Autodesk Inventor part; units mm, degrees
(part 2 of 2)
  circle A233 centre (35.381, -14.7938) radius 0.4555 projected
  circle A234 centre (37.921, -17.3338) radius 0.4555 projected
  circle A235 centre (35.381, -17.3338) radius 0.4555 projected
  circle A236 centre (35.381, -19.8738) radius 0.4555 projected
  circle A237 centre (35.381, -22.4138) radius 0.4555 projected
  circle A238 centre (37.921, -19.8738) radius 0.4555 projected
  circle A239 centre (37.921, -24.9538) radius 0.4555 projected
  circle A240 centre (37.921, -22.4138) radius 0.4555 projected
  circle A241 centre (35.381, -24.9538) radius 0.4555 projected
  circle A242 centre (37.921, -27.4938) radius 0.4555 projected
  circle A243 centre (35.381, -27.4938) radius 0.4555 projected
  circle A244 centre (37.921, -30.0338) radius 0.4555 projected
  circle A245 centre (35.381, -30.0338) radius 0.4555 projected
  circle A246 centre (37.921, -32.5738) radius 0.4555 projected
  circle A247 centre (35.381, -32.5738) radius 0.4555 projected
  circle A248 centre (37.921, -35.1138) radius 0.4555 projected
  circle A249 centre (35.381, -35.1138) radius 0.4555 projected
  circle A250 centre (35.381, -37.6538) radius 0.4555 projected
  circle A251 centre (81.101, -12.2538) radius 0.4555 projected
  circle A252 centre (78.561, -32.5738) radius 0.4555 projected
  circle A253 centre (81.101, -32.5738) radius 0.4555 projected
  circle A254 centre (78.561, -30.0338) radius 0.4555 projected
  circle A255 centre (81.101, -30.0338) radius 0.4555 projected
  circle A256 centre (78.561, -27.4938) radius 0.4555 projected
  circle A257 centre (81.101, -27.4938) radius 0.4555 projected
  circle A258 centre (78.561, -24.9538) radius 0.4555 projected
  circle A259 centre (81.101, -24.9538) radius 0.4555 projected
  circle A260 centre (78.561, -22.4138) radius 0.4555 projected
  circle A261 centre (81.101, -22.4138) radius 0.4555 projected
  circle A262 centre (78.561, -19.8738) radius 0.4555 projected
  circle A263 centre (81.101, -19.8738) radius 0.4555 projected
  circle A264 centre (78.561, -17.3338) radius 0.4555 projected
  circle A265 centre (81.101, -17.3338) radius 0.4555 projected
  circle A266 centre (78.561, -14.7938) radius 0.4555 projected
  circle A267 centre (81.101, -14.7938) radius 0.4555 projected
  circle A268 centre (78.561, -12.2538) radius 0.4555 projected
  circle A269 centre (78.561, -9.7138) radius 0.4555 projected
  circle A270 centre (81.101, -9.7138) radius 0.4555 projected
  circle A271 centre (78.561, -7.1738) radius 0.4555 projected
  circle A272 centre (81.101, -7.1738) radius 0.4555 projected
  circle A273 centre (78.561, -4.6338) radius 0.4555 projected
  circle A274 centre (81.101, -4.6338) radius 0.4555 projected
  circle A275 centre (78.561, -2.0938) radius 0.4555 projected
  circle A276 centre (81.101, -2.0938) radius 0.4555 projected
  circle A277 centre (78.561, 0.4462) radius 0.4555 projected
  circle A278 centre (81.101, 0.4462) radius 0.4555 projected
  circle A279 centre (78.561, 2.9862) radius 0.4555 projected
  circle A280 centre (81.101, 2.9862) radius 0.4555 projected
  circle A281 centre (78.561, 5.5262) radius 0.4555 projected
  circle A282 centre (81.101, 5.5262) radius 0.4555 projected
  circle A283 centre (81.101, 8.0662) radius 0.4555 projected
  circle A284 centre (78.561, 10.6062) radius 0.4555 projected
  circle A285 centre (81.101, 10.6062) radius 0.4555 projected
  circle A286 centre (78.561, 8.0662) radius 0.4555 projected
  circle A287 centre (2.0843, -29.8938) radius 0.91
  circle A288 centre (2.0843, -50.9442) radius 0.91
  circle A289 centre (44.0555, -71.8667) radius 0.91
  circle A290 centre (86.061, -50.8938) radius 0.91
  circle A291 centre (86.061, -29.8938) radius 0.91
  circle A292 centre (86.061, -8.8686) radius 0.91
  dimension "d27" = 1.82
  dimension "d28" = 1.82
  dimension "d29" = 1.82
  dimension "d30" = 1.82
  dimension "d31" = 1.82
  dimension "d32" = 1.82
  constraints: 6 centre point
  measures "d27" diameter of A287
  measures "d28" diameter of A288
  measures "d29" diameter of A289
  measures "d30" diameter of A290
  measures "d31" diameter of A291
  measures "d32" diameter of A292
extrude "Extrusion4" add sketch "Sketch4" along normal blind 3 contours A287 | A289 | A290 | A291 | A292
chamfer "Chamfer1" distance 3.5 angle 45 7 edges at (-0.0226, -39.7451, 10) (-36.0226, -39.7451, 10) (-39.6612, -21.0282, 10) (-39.8616, -0.0282, 10) (-39.6612, 21.1023, 10) (39.8358, 28.0032, 10) (39.8025, -0.0168, 10)
fillet "Fillet1" radius 0.5 14 edges at (-39.6612, 23.0023, 3.25) (-39.8616, 1.8718, 3.25) (-39.6612, -19.1282, 3.25) (-34.1226, -39.7451, 3.25) (-37.9226, -39.7451, 3.25) (1.8774, -39.7451, 3.25) (-1.9226, -39.7451, 3.25) (39.8358, 29.8938, 3.25) (39.8025, 1.8832, 3.25) (39.8025, -1.9168, 3.25) (39.8358, 26.1126, 3.25) (-39.6612, -22.9282, 3.25) (-39.8616, -1.9282, 3.25) (-39.6612, 19.2023, 3.25)
fillet "Fillet2" radius 5 8 edges at (41.5, -41.5, 26) (41.5, 41.5, 26) (-41.5, 41.5, 26) (-41.5, -41.5, 26) (-46.5, -46.5, 26) (46.5, -46.5, 26) (46.5, 46.5, 26) (-46.5, 46.5, 26)
body "Solid1"
